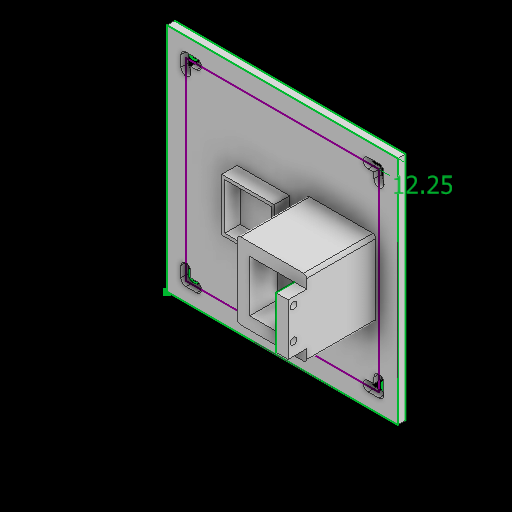
# Autodesk Inventor part: yield_bed
Saved by Autodesk Inventor 2025.1 (Build 291241000, 241)
## iProperties
Created: 2024-08-22
Part Number: yield_bed
Material: 일반
Document SubType Name: Modeling
Designer: ojs08
Density: 1 g/cm^3
Appearance: 기본값
Author: ojs08
Autodesk Inventor part; units mm, degrees
ref_plane "YZ Plane" through (0, 0, 0) normal (1, 0, 0) x (0, 1, 0)
ref_plane "XZ Plane" through (0, 0, 0) normal (0, 1, 0) x (-1, 0, 0)
ref_plane "XY Plane" through (0, 0, 0) normal (0, 0, 1) x (1, 0, 0)
sketch "스케치1" plane through (0, 0, 0) normal (0, 0, 1) x (1, 0, 0)
  line L0 (0, 150) -> (150, 150)
  line L1 (150, 150) -> (150, 0)
  line L2 (150, 0) -> (0, 0)
  line L3 (0, 0) -> (0, 150)
  dimension "d0" = 150
  dimension "d1" = 150
  constraints: 8 end point, 2 parallel, 1 coincident, 1 horizontal, 1 perpendicular
  measures "d0" distance of L0.start L0.end
  measures "d1" distance of L0.end L1.end
extrude "돌출1" add sketch "스케치1" along normal blind 5
sketch "스케치2" plane through (0, 0, 5) normal (0, 0, 1) x (1, 0, 0)
  line L0 (0, 0) -> (150, 0) projected
  line L1 (150, 0) -> (150, 150) projected
  line L2 (150, 150) -> (0, 150) projected
  line L3 (0, 150) -> (0, 0) projected
  line L4 (12.25, 137.75) -> (137.75, 137.75)
  line L5 (137.75, 137.75) -> (137.75, 12.25)
  line L6 (137.75, 12.25) -> (12.25, 12.25)
  line L7 (12.25, 12.25) -> (12.25, 137.75)
  dimension "d4" = 12.25
  constraints: 8 end point, 3 other
  measures "d4" distance between parallel lines of L4 L2
sketch "스케치4" plane through (0, 0, 0) normal (0, 0, -1) x (-1, 0, 0)
  line L0 (0, 0) -> (-150, 0) projected
  line L1 (0, 150) -> (0, 0) projected
  line L2 (-150, 150) -> (0, 150) projected
  line L3 (-150, 0) -> (-150, 150) projected
  line L4 (-12.25, 12.25) -> (-137.75, 12.25)
  line L5 (-137.75, 12.25) -> (-137.75, 137.75)
  line L6 (-137.75, 137.75) -> (-12.25, 137.75)
  line L7 (-12.25, 137.75) -> (-12.25, 12.25)
  circle A0 centre (-12.25, 137.75) radius 3.25
  circle A1 centre (-137.75, 137.75) radius 3.25
  circle A2 centre (-12.25, 12.25) radius 3.25
  circle A3 centre (-137.75, 12.25) radius 3.25
  line L8 (-12.25, 137.75) -> (-12.25, 130.75) construction
  line L9 (-9, 137.75) -> (-9, 130.75)
  line L10 (-15.5, 130.75) -> (-15.5, 137.75)
  arc A4 (-9, 137.75) -> (-15.5, 137.75) centre (-12.25, 137.75) ccw
  arc A5 (-15.5, 130.75) -> (-9, 130.75) centre (-12.25, 130.75) ccw
  line L11 (-12.25, 137.75) -> (-19.25, 137.75) construction
  line L12 (-12.25, 141.0002) -> (-19.25, 141.0002)
  line L13 (-19.25, 134.4998) -> (-12.25, 134.4998)
  arc A6 (-12.25, 134.4998) -> (-12.25, 141.0002) centre (-12.25, 137.75) ccw
  arc A7 (-19.25, 141.0002) -> (-19.25, 134.4998) centre (-19.25, 137.75) ccw
  point P0 (-12.25, 134.25)
  point P1 (-15.75, 137.75)
  dimension "d22" = 12.25
  dimension "d23" = 6.5
  dimension "d26" = 125.5
  dimension "d33" = 125.5
  dimension "d57" = 7
  dimension "d58" = 7
  constraints: 24 end point, 8 centre point, 8 point on circle, 8 tangent, 2 midpoint, 2 parallel, 2 point on line, 1 coincident, 1 horizontal, 1 vertical, 9 other
  measures "d22" distance between parallel lines of L6 L2
  measures "d23" diameter of A0
  measures "d26" distance of L8.start A1.centre
  measures "d33" distance of L8.start A2.centre
  measures "d57" distance of L9.start L9.end
  measures "d58" distance of L13.start L13.end
extrude "돌출3" cut sketch "스케치4" against normal blind 3.5 contours A3 L5 L4 | L4 L5 A3 | A2 L7 L4 | L4 L7 A2 | A1 L6 L5 | L5 L6 A1 | A0 L6 L7 | L7 L6 A0
sketch "스케치8" plane through (0, 0, 5) normal (0, 0, 1) x (1, 0, 0)
  point P0 (0, 0)
sketch "스케치9" plane through (0, 0, 0) normal (0, 0, -1) x (-1, 0, 0)
  point P0 (0, 0)
sketch "스케치10" plane through (0, 0, 0) normal (0, 0, -1) x (-1, 0, 0)
  circle A0 centre (-12.25, 137.75) radius 3.25 projected
  circle A1 centre (-137.75, 137.75) radius 3.25 projected
  circle A2 centre (-137.75, 12.25) radius 3.25 projected
  circle A3 centre (-12.25, 12.25) radius 3.25 projected
  circle A4 centre (-137.75, 12.25) radius 3.25 projected
  circle A5 centre (-12.25, 12.25) radius 3.25 projected
  circle A6 centre (-137.75, 137.75) radius 3.25 projected
  circle A7 centre (-12.25, 137.75) radius 3.25 projected
  line L0 (0, 0) -> (-150, 0) projected
  line L1 (0, 150) -> (0, 0) projected
  line L2 (-150, 150) -> (0, 150) projected
  line L3 (-150, 0) -> (-150, 150) projected
sketch "스케치11" plane through (0, 0, 0) normal (0, 0, -1) x (-1, 0, 0)
  circle A0 centre (-12.25, 137.75) radius 3.25 projected
  line L0 (-12.25, 137.75) -> (-12.25, 130.75) construction
  line L1 (-9, 137.75) -> (-9, 130.75)
  line L2 (-15.5, 130.75) -> (-15.5, 137.75)
  arc A1 (-9, 137.75) -> (-15.5, 137.75) centre (-12.25, 137.75) ccw
  arc A2 (-15.5, 130.75) -> (-9, 130.75) centre (-12.25, 130.75) ccw
  line L3 (-12.25, 137.75) -> (-19.25, 137.75) construction
  line L4 (-12.25, 141) -> (-19.25, 141)
  line L5 (-19.25, 134.5) -> (-12.25, 134.5)
  arc A3 (-12.25, 134.5) -> (-12.25, 141) centre (-12.25, 137.75) ccw
  arc A4 (-19.25, 141) -> (-19.25, 134.5) centre (-19.25, 137.75) ccw
  point P0 (0, 0)
  point P1 (-12.25, 134.25)
  point P2 (-15.75, 137.75)
  point P3 (-15.5, 134.5)
  dimension "d60" = 3.25
  dimension "d61" = 7
  dimension "d62" = 7
  dimension "d63" = 3.25
  constraints: 16 end point, 8 point on circle, 8 tangent, 4 centre point, 2 midpoint, 2 parallel, 1 perpendicular, 1 vertical
  measures "d60" radius of A3
  measures "d61" distance of L5.start L5.end
  measures "d62" distance of L2.start L2.end
  measures "d63" radius of A2
extrude "돌출7" cut sketch "스케치11" against normal blind 5
sketch "스케치12" plane through (0, 0, 0) normal (0, 0, -1) x (-1, 0, 0)
  circle A0 centre (-12.25, 12.25) radius 3.25 projected
  line L0 (-12.25, 12.25) -> (-12.25, 19.25) construction
  line L1 (-9, 12.25) -> (-9, 19.25)
  line L2 (-15.5, 19.25) -> (-15.5, 12.25)
  arc A1 (-15.5, 12.25) -> (-9, 12.25) centre (-12.25, 12.25) ccw
  arc A2 (-9, 19.25) -> (-15.5, 19.25) centre (-12.25, 19.25) ccw
  line L3 (-12.25, 12.25) -> (-19.25, 12.25) construction
  line L4 (-12.25, 15.5) -> (-19.25, 15.5)
  line L5 (-19.25, 9) -> (-12.25, 9)
  arc A3 (-12.25, 9) -> (-12.25, 15.5) centre (-12.25, 12.25) ccw
  arc A4 (-19.25, 15.5) -> (-19.25, 9) centre (-19.25, 12.25) ccw
  line L6 (-137.75, 12.25) -> (-137.75, 19.25) construction
  line L7 (-134.5, 12.25) -> (-134.5, 19.25)
  line L8 (-141, 19.25) -> (-141, 12.25)
  arc A5 (-141, 12.25) -> (-134.5, 12.25) centre (-137.75, 12.25) ccw
  arc A6 (-134.5, 19.25) -> (-141, 19.25) centre (-137.75, 19.25) ccw
  line L9 (-137.75, 12.25) -> (-130.75, 12.25) construction
  line L10 (-137.75, 15.5) -> (-130.75, 15.5)
  line L11 (-130.75, 9) -> (-137.75, 9)
  arc A7 (-137.75, 15.5) -> (-137.75, 9) centre (-137.75, 12.25) ccw
  arc A8 (-130.75, 9) -> (-130.75, 15.5) centre (-130.75, 12.25) ccw
  circle A9 centre (-137.75, 137.75) radius 3.25 projected
  line L12 (-137.75, 137.75) -> (-137.75, 130.75) construction
  line L13 (-134.5, 137.75) -> (-134.5, 130.75)
  line L14 (-141, 130.75) -> (-141, 137.75)
  arc A10 (-134.5, 137.75) -> (-141, 137.75) centre (-137.75, 137.75) ccw
  arc A11 (-141, 130.75) -> (-134.5, 130.75) centre (-137.75, 130.75) ccw
  line L15 (-137.75, 137.75) -> (-130.75, 137.75) construction
  line L16 (-137.75, 134.5) -> (-130.75, 134.5)
  line L17 (-130.75, 141) -> (-137.75, 141)
  arc A12 (-137.75, 141) -> (-137.75, 134.5) centre (-137.75, 137.75) ccw
  arc A13 (-130.75, 134.5) -> (-130.75, 141) centre (-130.75, 137.75) ccw
  point P0 (0, 0)
  point P1 (-12.25, 15.75)
  point P2 (-15.75, 12.25)
  point P3 (-137.75, 15.75)
  point P4 (-134.25, 12.25)
  point P5 (-137.75, 134.25)
  point P6 (-134.25, 137.75)
  point P7 (-134.5, 134.5)
  point P8 (-134.5, 15.5)
  point P9 (-15.5, 15.5)
  dimension "d66" = 3.25
  dimension "d67" = 7
  dimension "d68" = 7
  dimension "d69" = 3.25
  dimension "d70" = 3.25
  dimension "d71" = 7
  dimension "d72" = 3.25
  dimension "d73" = 7
  dimension "d74" = 3.25
  dimension "d75" = 3.25
  dimension "d76" = 7
  dimension "d77" = 7
  constraints: 48 end point, 24 point on circle, 24 tangent, 12 centre point, 6 midpoint, 6 parallel, 3 vertical, 2 horizontal, 1 perpendicular
  measures "d66" radius of A4
  measures "d67" distance of L2.start L2.end
  measures "d68" distance of L5.start L5.end
  measures "d69" radius of A2
  measures "d70" radius of A8
  measures "d71" distance of L11.start L11.end
  measures "d72" radius of A6
  measures "d73" distance of L8.start L8.end
  measures "d74" radius of A11
  measures "d75" radius of A13
  measures "d76" distance of L14.start L14.end
  measures "d77" distance of L16.start L16.end
extrude "돌출8" cut sketch "스케치12" against normal blind 5
sketch "스케치13" plane through (0, 0, 5) normal (0, 0, 1) x (1, 0, 0)
  line L0 (90.75, 99.75) -> (90.75, 50.25) projected
  line L1 (90.75, 50.25) -> (135.75, 50.25) projected
  line L2 (135.75, 99.75) -> (90.75, 99.75) projected
  line L3 (135.75, 99.75) -> (135.75, 50.25) projected
  point P0 (0, 0)
extrude "돌출9" add sketch "스케치13" along normal blind 27
sketch "스케치14" plane through (0, 0, 32) normal (0, 0, 1) x (1, 0, 0)
  line L0 (90.75, 99.75) -> (90.75, 50.25) projected
  line L1 (90.75, 50.25) -> (135.75, 50.25) projected
  line L2 (135.75, 50.25) -> (135.75, 99.75) projected
  line L3 (135.75, 99.75) -> (90.75, 99.75) projected
  line L4 (127.75, 58.25) -> (98.75, 58.25)
  line L5 (98.75, 58.25) -> (98.75, 91.75)
  line L6 (98.75, 91.75) -> (127.75, 91.75)
  line L7 (127.75, 91.75) -> (127.75, 58.25)
  point P0 (0, 0)
  dimension "d84" = 8
  constraints: 8 end point, 3 other
  measures "d84" distance between parallel lines of L1 L4
extrude "돌출10" add sketch "스케치14" along normal blind 18
sketch "스케치15" plane through (0, 0, 50) normal (0, 0, 1) x (1, 0, 0)
  line L0 (127.75, 91.75) -> (127.75, 58.25) projected
  line L1 (127.75, 58.25) -> (135.75, 58.25)
  line L2 (135.75, 99.75) -> (135.75, 50.25) projected
  line L3 (127.75, 91.75) -> (135.75, 91.75)
  point P0 (0, 0)
  constraints: 4 end point, 2 point on line, 1 horizontal, 1 perpendicular
extrude "돌출11" add sketch "스케치15" along normal blind 12
sketch "스케치16" plane through (127.75, 58.25, 32) normal (-1, 0, 0) x (0, 0, 1)
  line L0 (0, 0) -> (0, 33.5) projected
  line L1 (0, 0) -> (0, 33.5) projected
  line L2 (0, 0) -> (18, 0) projected
  line L3 (18, 0) -> (30, 0) projected
  line L4 (30, 33.5) -> (30, 0) projected
  line L5 (18, 33.5) -> (30, 33.5) projected
  line L6 (0, 33.5) -> (18, 33.5) projected
  point P0 (-32, -58.25)
sketch "스케치17" plane through (135.75, 50.25, 5) normal (1, 0, 0) x (0, 0, -1)
  point P0 (5, -50.25)
sketch "스케치18" plane through (127.75, 58.25, 32) normal (-1, 0, 0) x (0, 0, 1)
  circle A0 centre (26.5, 28.5) radius 2.2
  circle A1 centre (26.5, 8.5) radius 2.2
  line L0 (18, 33.5) -> (30, 33.5) projected
  line L1 (0, 0) -> (0, 33.5) projected
  point P0 (-32, -58.25)
  dimension "d89" = 4.4
  dimension "d90" = 5
  dimension "d91" = 26.5
  dimension "d92" = 26.5
  dimension "d93" = 20
  dimension "d94" = 4.4
  constraints: 2 centre point
  measures "d89" diameter of A0
  measures "d90" distance from line of L0 A0.centre
  measures "d91" distance from line of L1 A0.centre
  measures "d92" distance from line of L1 A1.centre
  measures "d93" distance of A0.centre A1.centre
  measures "d94" diameter of A1
extrude "돌출12" cut sketch "스케치18" against normal blind 8
sketch "스케치19" plane through (0, 0, 5) normal (0, 0, 1) x (1, 0, 0)
  point P0 (0, 0)
fillet "모깎기3" radius 2 8 edges at (90.75, 99.75, 41) (90.75, 99.75, 18.5) (135.75, 99.75, 41) (135.75, 99.75, 18.5) (90.75, 50.25, 41) (90.75, 50.25, 18.5) (135.75, 50.25, 41) (135.75, 50.25, 18.5)
sketch "스케치20" plane through (0, 0, 5) normal (0, 0, 1) x (1, 0, 0)
  line L0 (77.75, 61.65) -> (47.55, 61.65)
  line L1 (47.55, 61.65) -> (47.55, 91.85)
  line L2 (47.55, 91.85) -> (77.75, 91.85)
  line L3 (77.75, 91.85) -> (77.75, 61.65)
  line L4 (137.75, 12.25) -> (12.25, 12.25) projected
  line L5 (90.75, 97.75) -> (90.75, 52.25) projected
  line L6 (45.55, 59.65) -> (79.75, 59.65)
  line L7 (79.75, 59.65) -> (79.75, 93.85)
  line L8 (79.75, 93.85) -> (45.55, 93.85)
  line L9 (45.55, 93.85) -> (45.55, 59.65)
  line L10 (90.75, 52.25) -> (90.75, 97.75) projected
  point P0 (0, 0)
  point P1 (90.75, 57.9)
  point P2 (90.75, 92.1)
  dimension "d98" = 30.2
  dimension "d99" = 30.2
  dimension "d100" = 49.4
  dimension "d101" = 2
  dimension "d104" = 11
  constraints: 16 end point, 4 parallel, 2 perpendicular, 1 horizontal, 3 other
  measures "d98" distance of L0.start L0.end
  measures "d99" distance of L0.end L1.end
  measures "d100" distance between parallel lines of L0 L4
  measures "d101" distance between parallel lines of L6 L0
  measures "d104" distance between parallel lines of L5 L7
extrude "돌출13" add sketch "스케치20" along normal blind 10
